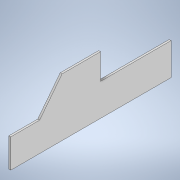
# Autodesk Inventor part: zijkant
Saved by Autodesk Inventor 2022 (Build 260153000, 153)
## iProperties
Created: 2021-12-16
Part Number: zijkant
Material: Generic
Document SubType Name: Modeling
Designer: keemi
Density: 1 g/cm^3
Appearance: Default
Author: keemi
Autodesk Inventor part; units mm, degrees
ref_plane "YZ Plane" through (0, 0, 0) normal (1, 0, 0) x (0, 1, 0)
ref_plane "XZ Plane" through (0, 0, 0) normal (0, 1, 0) x (-1, 0, 0)
ref_plane "XY Plane" through (0, 0, 0) normal (0, 0, 1) x (1, 0, 0)
sketch "Sketch1" plane through (0, 0, 0) normal (1, 0, 0) x (0, 1, 0)
  line L0 (0, 0) -> (0, -250)
  line L1 (0, -250) -> (50, -250)
  line L2 (50, -250) -> (50, -140)
  line L3 (50, -140) -> (90, -140)
  line L4 (90, -140) -> (90, -80)
  line L5 (90, -80) -> (157.3677, -80) construction
  line L6 (90, -80) -> (146.3502, -80) construction
  line L7 (46.4138, 0) -> (0, 0)
  line L8 (90, -80) -> (146.8977, -80) construction
  line L9 (0, -43.4268) -> (0, 0)
  line L10 (0, 0) -> (46.4138, 0)
  line L11 (0, 0) -> (45, 0)
  line L12 (0, 0) -> (45, 0) construction
  line L13 (45, 0) -> (45, -45)
  line L14 (45, -45) -> (90, -80)
  dimension "d0" = 250
  dimension "d1" = 50
  dimension "d2" = 110
  dimension "d3" = 40
  dimension "d4" = 60
  dimension "d8" = 45
  dimension "d9" = 0
  dimension "d10" = 45
  constraints: 30 end point, 5 horizontal, 4 perpendicular, 1 collinear, 1 parallel, 1 vertical
  measures "d0" distance of L0.start L0.end
  measures "d1" distance of L0.end L1.end
  measures "d2" distance of L1.end L2.end
  measures "d3" distance of L2.end L3.end
  measures "d4" distance of L3.end L4.end
  measures "d8" distance of L0.start L11.end
  measures "d9" distance between parallel lines of L11 L12
  measures "d10" distance of L11.end L13.end
extrude "Extrusion1" add sketch "Sketch1" along normal blind 3
body "Solid1"
